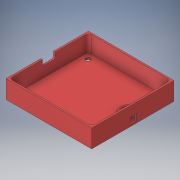
# Autodesk Inventor part: BOTTOM
Saved by Autodesk Inventor 2019 (Build 230136000, 136)
## iProperties
Created: 2018-12-19
Part Number: BOTTOM
Material: Типовые
Document SubType Name: Modeling
Designer: aldanstar
Density: 1 g/cm^3
Appearance: По умолчанию
Author: aldanstar
Autodesk Inventor part; units mm, degrees
ref_plane "YZ Plane" through (0, 0, 0) normal (1, 0, 0) x (0, 1, 0)
ref_plane "XZ Plane" through (0, 0, 0) normal (0, 1, 0) x (-1, 0, 0)
ref_plane "XY Plane" through (0, 0, 0) normal (0, 0, 1) x (1, 0, 0)
sketch "Эскиз1" plane through (0, 0, 0) normal (0, 1, 0) x (-1, 0, 0)
  line L0 (26, 25) -> (-26, 25)
  line L1 (-26, 25) -> (-26, -25)
  line L2 (-26, -25) -> (26, -25)
  line L3 (26, -25) -> (26, 25)
  line L4 (36.4, 0) -> (-36.4, 0) projected
  line L5 (0, -35) -> (0, 35) projected
  point P0 (0, 0)
  dimension "d0" = 52
  dimension "d1" = 50
  constraints: 8 end point, 2 parallel, 1 horizontal, 1 perpendicular, 2 other
  measures "d0" distance of L1.end L2.end
  measures "d1" distance of L2.end L0.start
extrude "Выдавливание1" add sketch "Эскиз1" along normal blind 11
shell "Оболочка1" thickness 1 removed faces 1 at (-8.6667, 11, -8.3333)
sketch "Эскиз2" plane through (-26, 0, -25) normal (-1, 0, 0) x (0, 0, 1)
  line L0 (28.9, 7.4) -> (21.1, 7.4)
  line L1 (21.1, 7.4) -> (21.1, 11)
  line L2 (21.1, 11) -> (28.9, 11)
  line L3 (28.9, 11) -> (28.9, 7.4)
  line L4 (0, 0) -> (50, 0) projected
  line L5 (25, -2.2) -> (25, 13.2) projected
  line L6 (0, 11) -> (50, 11) projected
  point P0 (25, 0)
  dimension "d5" = 7.4
  dimension "d7" = 7.8
  constraints: 8 end point, 2 parallel, 1 collinear, 1 horizontal, 1 perpendicular, 1 other
  measures "d5" distance between parallel lines of L4 L0
  measures "d7" distance of L0.start L0.end
extrude "Выдавливание2" cut sketch "Эскиз2" against normal up to surface (1 mm away)
fillet "Сопряжение1" radius 1.5 2 edges at (-25.5, 7.4, -3.9) (-25.5, 7.4, 3.9)
fillet "Сопряжение2" radius 2 4 edges at (25, 6, 24) (25, 6, -24) (-25, 6, -24) (-25, 6, 24)
sketch "Эскиз4" plane through (25, 1, -22) normal (-1, 0, 0) x (0, 0, 1)
  line L0 (44, 0) -> (0, 0) projected
  line L1 (24, 0) -> (20, 0)
  line L2 (20, 0) -> (20, 4)
  line L3 (20, 4) -> (24, 4)
  line L4 (24, 4) -> (24, 0)
  line L5 (22, -3.2) -> (22, 12.2) projected
  point P0 (22, -1)
  dimension "d16" = 4
  dimension "d17" = 4
  constraints: 8 end point, 2 parallel, 1 horizontal, 1 perpendicular, 1 point on line, 1 other
  measures "d16" distance of L2.end L3.end
  measures "d17" distance of L3.end L1.start
extrude "Выдавливание4" cut sketch "Эскиз4" against normal through all
sketch "Эскиз5" plane through (-23, 1, 24) normal (0, 1, 0) x (1, 0, 0)
  line L0 (48, 26) -> (48, 22) construction
  circle A0 centre (48, 24) radius 7 construction
  line L1 (48, 26) -> (48, 46) construction
  line L2 (48, 26.75) -> (41, 26.75) construction
  line L3 (41, 26.75) -> (41, 21.25) construction
  line L4 (41, 21.25) -> (48, 21.25) construction
  line L5 (48, 21.25) -> (48, 26.75) construction
  line L6 (-14.64, 24) -> (66.84, 24) construction
  line L7 (48, 2) -> (48, 22) construction
  line L8 (41, 21.25) -> (48, 21.25) construction
  line L9 (48, 21.25) -> (48, 20.25) construction
  line L10 (48, 20.25) -> (41, 20.25) construction
  line L11 (41, 20.25) -> (41, 21.25) construction
  line L12 (41, 26.75) -> (48, 26.75) construction
  line L13 (48, 26.75) -> (48, 27.75) construction
  line L14 (48, 27.75) -> (41, 27.75) construction
  line L15 (41, 27.75) -> (41, 26.75) construction
  arc A1 (42.1104, 21.25) -> (42.6908, 20.25) centre (48, 24) ccw
  arc A2 (42.6908, 27.75) -> (42.1104, 26.75) centre (48, 24) ccw
  arc A3 (42.1104, 26.75) -> (42.1104, 21.25) centre (48, 24) ccw
  arc A4 (43.2369, 26.75) -> (43.2369, 21.25) centre (48, 24) ccw
  line L16 (43.2369, 26.75) -> (48, 26.75)
  line L17 (48, 26.75) -> (48, 27.75)
  line L18 (48, 27.75) -> (42.6908, 27.75)
  line L19 (43.2369, 21.25) -> (48, 21.25)
  line L20 (48, 21.25) -> (48, 20.25)
  line L21 (42.6908, 20.25) -> (48, 20.25)
  point P0 (23, 24)
  dimension "d20" = 14
  dimension "d21" = 5.5
  dimension "d22" = 1
  dimension "d23" = 1
  dimension "d24" = 0.5
  dimension "d25" = 1
  constraints: 36 end point, 9 point on line, 8 point on circle, 7 parallel, 5 centre point, 4 collinear, 4 perpendicular, 3 coincident, 3 horizontal, 2 midpoint, 1 concentric, 1 tangent, 1 other
  measures "d20" diameter of A0
  measures "d21" distance between parallel lines of L2 L4
  measures "d22" distance between parallel lines of L4 L10
  measures "d23" distance between parallel lines of L2 L14
  measures "d24" radial gap between concentric circles of A1 A0
  measures "d25" radial gap between concentric circles of A4 A3
extrude "Выдавливание5" add sketch "Эскиз5" along normal blind 5
sketch "Эскиз8" plane through (-23, 1, -24) normal (0, 1, 0) x (1, 0, 0)
  line L0 (1.875, -4.025) -> (44.125, -4.025) construction
  line L1 (44.125, -4.025) -> (44.125, -43.975) construction
  line L2 (44.125, -43.975) -> (1.875, -43.975) construction
  line L3 (1.875, -43.975) -> (1.875, -4.025) construction
  line L4 (23, 11) -> (23, -59) construction
  line L5 (-13.4, -24) -> (59.4, -24) construction
  circle A0 centre (1.875, -4.025) radius 1.35
  circle A1 centre (44.125, -4.025) radius 1.35
  circle A2 centre (1.875, -43.975) radius 1.35
  circle A3 centre (44.125, -43.975) radius 1.35
  point P0 (23, -24)
  dimension "d33" = 42.25
  dimension "d34" = 39.95
  dimension "d35" = 2.7
  constraints: 8 end point, 4 centre point, 4 coincident, 3 equal radius, 2 parallel, 1 horizontal, 1 perpendicular, 1 point on line, 2 other
  measures "d33" distance of L0.start L0.end
  measures "d34" distance of L0.end L1.end
  measures "d35" diameter of A0
extrude "Выдавливание7" cut sketch "Эскиз8" against normal through all
